Autodesk Fusion 360 part; units mm, degrees
(part 11 of 12)
  line L1843 (137.546, 134.2487) -> (141.8762, 136.7487)
  line L1844 (141.8762, 136.7487) -> (141.8762, 141.7487)
  line L1845 (141.8762, 141.7487) -> (137.546, 144.2487)
  line L1846 (148.2063, 144.2487) -> (143.8762, 141.7487)
  line L1847 (143.8762, 141.7487) -> (143.8762, 136.7487)
  line L1848 (143.8762, 136.7487) -> (148.2063, 134.2487)
  line L1849 (148.2063, 134.2487) -> (152.5364, 136.7487)
  line L1850 (152.5364, 136.7487) -> (152.5364, 141.7487)
  line L1851 (152.5364, 141.7487) -> (148.2063, 144.2487)
  line L1852 (-59.6687, 153.4808) -> (-63.9988, 150.9808)
  line L1853 (-63.9988, 150.9808) -> (-63.9988, 145.9808)
  line L1854 (-63.9988, 145.9808) -> (-59.6687, 143.4808)
  line L1855 (-59.6687, 143.4808) -> (-55.3385, 145.9808)
  line L1856 (-55.3385, 145.9808) -> (-55.3385, 150.9808)
  line L1857 (-55.3385, 150.9808) -> (-59.6687, 153.4808)
  line L1858 (-49.0084, 153.4808) -> (-53.3385, 150.9808)
  line L1859 (-53.3385, 150.9808) -> (-53.3385, 145.9808)
  line L1860 (-53.3385, 145.9808) -> (-49.0084, 143.4808)
  line L1861 (-49.0084, 143.4808) -> (-44.6783, 145.9808)
  line L1862 (-44.6783, 145.9808) -> (-44.6783, 150.9808)
  line L1863 (-44.6783, 150.9808) -> (-49.0084, 153.4808)
  line L1864 (-38.3482, 153.4808) -> (-42.6783, 150.9808)
  line L1865 (-42.6783, 150.9808) -> (-42.6783, 145.9808)
  line L1866 (-42.6783, 145.9808) -> (-38.3482, 143.4808)
  line L1867 (-38.3482, 143.4808) -> (-34.018, 145.9808)
  line L1868 (-34.018, 145.9808) -> (-34.018, 150.9808)
  line L1869 (-34.018, 150.9808) -> (-38.3482, 153.4808)
  line L1870 (-27.6879, 153.4808) -> (-32.018, 150.9808)
  line L1871 (-32.018, 150.9808) -> (-32.018, 145.9808)
  line L1872 (-32.018, 145.9808) -> (-27.6879, 143.4808)
  line L1873 (-27.6879, 143.4808) -> (-23.3578, 145.9808)
  line L1874 (-23.3578, 145.9808) -> (-23.3578, 150.9808)
  line L1875 (-23.3578, 150.9808) -> (-27.6879, 153.4808)
  line L1876 (-17.0277, 153.4808) -> (-21.3578, 150.9808)
  line L1877 (-21.3578, 150.9808) -> (-21.3578, 145.9808)
  line L1878 (-21.3578, 145.9808) -> (-17.0277, 143.4808)
  line L1879 (-17.0277, 143.4808) -> (-12.6975, 145.9808)
  line L1880 (-12.6975, 145.9808) -> (-12.6975, 150.9808)
  line L1881 (-12.6975, 150.9808) -> (-17.0277, 153.4808)
  line L1882 (-6.3674, 153.4808) -> (-10.6975, 150.9808)
  line L1883 (-10.6975, 150.9808) -> (-10.6975, 145.9808)
  line L1884 (-10.6975, 145.9808) -> (-6.3674, 143.4808)
  line L1885 (-6.3674, 143.4808) -> (-2.0373, 145.9808)
  line L1886 (-2.0373, 145.9808) -> (-2.0373, 150.9808)
  line L1887 (-2.0373, 150.9808) -> (-6.3674, 153.4808)
  line L1888 (4.2929, 153.4808) -> (-0.0373, 150.9808)
  line L1889 (-0.0373, 150.9808) -> (-0.0373, 145.9808)
  line L1890 (-0.0373, 145.9808) -> (4.2929, 143.4808)
  line L1891 (4.2929, 143.4808) -> (8.623, 145.9808)
  line L1892 (8.623, 145.9808) -> (8.623, 150.9808)
  line L1893 (8.623, 150.9808) -> (4.2929, 153.4808)
  line L1894 (14.9531, 153.4808) -> (10.623, 150.9808)
  line L1895 (10.623, 150.9808) -> (10.623, 145.9808)
  line L1896 (10.623, 145.9808) -> (14.9531, 143.4808)
  line L1897 (14.9531, 143.4808) -> (19.2832, 145.9808)
  line L1898 (19.2832, 145.9808) -> (19.2832, 150.9808)
  line L1899 (19.2832, 150.9808) -> (14.9531, 153.4808)
  line L1900 (25.6134, 153.4808) -> (21.2832, 150.9808)
  line L1901 (21.2832, 150.9808) -> (21.2832, 145.9808)
  line L1902 (21.2832, 145.9808) -> (25.6134, 143.4808)
  line L1903 (25.6134, 143.4808) -> (29.9435, 145.9808)
  line L1904 (29.9435, 145.9808) -> (29.9435, 150.9808)
  line L1905 (29.9435, 150.9808) -> (25.6134, 153.4808)
  line L1906 (36.2736, 153.4808) -> (31.9435, 150.9808)
  line L1907 (31.9435, 150.9808) -> (31.9435, 145.9808)
  line L1908 (31.9435, 145.9808) -> (36.2736, 143.4808)
  line L1909 (36.2736, 143.4808) -> (40.6037, 145.9808)
  line L1910 (40.6037, 145.9808) -> (40.6037, 150.9808)
  line L1911 (40.6037, 150.9808) -> (36.2736, 153.4808)
  line L1912 (46.9339, 153.4808) -> (42.6037, 150.9808)
  line L1913 (42.6037, 150.9808) -> (42.6037, 145.9808)
  line L1914 (42.6037, 145.9808) -> (46.9339, 143.4808)
  line L1915 (46.9339, 143.4808) -> (51.264, 145.9808)
  line L1916 (51.264, 145.9808) -> (51.264, 150.9808)
  line L1917 (51.264, 150.9808) -> (46.9339, 153.4808)
  line L1918 (57.5941, 153.4808) -> (53.264, 150.9808)
  line L1919 (53.264, 150.9808) -> (53.264, 145.9808)
  line L1920 (53.264, 145.9808) -> (57.5941, 143.4808)
  line L1921 (57.5941, 143.4808) -> (61.9242, 145.9808)
  line L1922 (61.9242, 145.9808) -> (61.9242, 150.9808)
  line L1923 (61.9242, 150.9808) -> (57.5941, 153.4808)
  line L1924 (68.2544, 153.4808) -> (63.9242, 150.9808)
  line L1925 (63.9242, 150.9808) -> (63.9242, 145.9808)
  line L1926 (63.9242, 145.9808) -> (68.2544, 143.4808)
  line L1927 (68.2544, 143.4808) -> (72.5845, 145.9808)
  line L1928 (72.5845, 145.9808) -> (72.5845, 150.9808)
  line L1929 (72.5845, 150.9808) -> (68.2544, 153.4808)
  line L1930 (78.9146, 153.4808) -> (74.5845, 150.9808)
  line L1931 (74.5845, 150.9808) -> (74.5845, 145.9808)
  line L1932 (74.5845, 145.9808) -> (78.9146, 143.4808)
  line L1933 (78.9146, 143.4808) -> (83.2448, 145.9808)
  line L1934 (83.2448, 145.9808) -> (83.2448, 150.9808)
  line L1935 (83.2448, 150.9808) -> (78.9146, 153.4808)
  line L1936 (89.5749, 153.4808) -> (85.2448, 150.9808)
  line L1937 (85.2448, 150.9808) -> (85.2448, 145.9808)
  line L1938 (85.2448, 145.9808) -> (89.5749, 143.4808)
  line L1939 (89.5749, 143.4808) -> (93.905, 145.9808)
  line L1940 (93.905, 145.9808) -> (93.905, 150.9808)
  line L1941 (93.905, 150.9808) -> (89.5749, 153.4808)
  line L1942 (100.2351, 153.4808) -> (95.905, 150.9808)
  line L1943 (95.905, 150.9808) -> (95.905, 145.9808)
  line L1944 (95.905, 145.9808) -> (100.2351, 143.4808)
  line L1945 (100.2351, 143.4808) -> (104.5653, 145.9808)
  line L1946 (104.5653, 145.9808) -> (104.5653, 150.9808)
  line L1947 (104.5653, 150.9808) -> (100.2351, 153.4808)
  line L1948 (110.8954, 153.4808) -> (106.5653, 150.9808)
  line L1949 (106.5653, 150.9808) -> (106.5653, 145.9808)
  line L1950 (106.5653, 145.9808) -> (110.8954, 143.4808)
  line L1951 (110.8954, 143.4808) -> (115.2255, 145.9808)
  line L1952 (115.2255, 145.9808) -> (115.2255, 150.9808)
  line L1953 (115.2255, 150.9808) -> (110.8954, 153.4808)
  line L1954 (121.5556, 153.4808) -> (117.2255, 150.9808)
  line L1955 (117.2255, 150.9808) -> (117.2255, 145.9808)
  line L1956 (117.2255, 145.9808) -> (121.5556, 143.4808)
  line L1957 (121.5556, 143.4808) -> (125.8858, 145.9808)
  line L1958 (125.8858, 145.9808) -> (125.8858, 150.9808)
  line L1959 (125.8858, 150.9808) -> (121.5556, 153.4808)
  line L1960 (132.2159, 153.4808) -> (127.8858, 150.9808)
  line L1961 (127.8858, 150.9808) -> (127.8858, 145.9808)
  line L1962 (127.8858, 145.9808) -> (132.2159, 143.4808)
  line L1963 (132.2159, 143.4808) -> (136.546, 145.9808)
  line L1964 (136.546, 145.9808) -> (136.546, 150.9808)
  line L1965 (136.546, 150.9808) -> (132.2159, 153.4808)
  line L1966 (142.8762, 153.4808) -> (138.546, 150.9808)
  line L1967 (138.546, 150.9808) -> (138.546, 145.9808)
  line L1968 (138.546, 145.9808) -> (142.8762, 143.4808)
  line L1969 (142.8762, 143.4808) -> (147.2063, 145.9808)
  line L1970 (147.2063, 145.9808) -> (147.2063, 150.9808)
  line L1971 (147.2063, 150.9808) -> (142.8762, 153.4808)
  line L1972 (-64.9988, 162.7128) -> (-69.3289, 160.2128)
  line L1973 (-69.3289, 160.2128) -> (-69.3289, 155.2128)
  line L1974 (-69.3289, 155.2128) -> (-64.9988, 152.7128)
  line L1975 (-64.9988, 152.7128) -> (-60.6687, 155.2128)
  line L1976 (-60.6687, 155.2128) -> (-60.6687, 160.2128)
  line L1977 (-60.6687, 160.2128) -> (-64.9988, 162.7128)
  line L1978 (-54.3385, 162.7128) -> (-58.6687, 160.2128)
  line L1979 (-58.6687, 160.2128) -> (-58.6687, 155.2128)
  line L1980 (-58.6687, 155.2128) -> (-54.3385, 152.7128)
  line L1981 (-54.3385, 152.7128) -> (-50.0084, 155.2128)
  line L1982 (-50.0084, 155.2128) -> (-50.0084, 160.2128)
  line L1983 (-50.0084, 160.2128) -> (-54.3385, 162.7128)
  line L1984 (-43.6783, 162.7128) -> (-48.0084, 160.2128)
  line L1985 (-48.0084, 160.2128) -> (-48.0084, 155.2128)
  line L1986 (-48.0084, 155.2128) -> (-43.6783, 152.7128)
  line L1987 (-43.6783, 152.7128) -> (-39.3482, 155.2128)
  line L1988 (-39.3482, 155.2128) -> (-39.3482, 160.2128)
  line L1989 (-39.3482, 160.2128) -> (-43.6783, 162.7128)
  line L1990 (-33.018, 162.7128) -> (-37.3482, 160.2128)
  line L1991 (-37.3482, 160.2128) -> (-37.3482, 155.2128)
  line L1992 (-37.3482, 155.2128) -> (-33.018, 152.7128)
  line L1993 (-33.018, 152.7128) -> (-28.6879, 155.2128)
  line L1994 (-28.6879, 155.2128) -> (-28.6879, 160.2128)
  line L1995 (-28.6879, 160.2128) -> (-33.018, 162.7128)
  line L1996 (-22.3578, 162.7128) -> (-26.6879, 160.2128)
  line L1997 (-26.6879, 160.2128) -> (-26.6879, 155.2128)
  line L1998 (-26.6879, 155.2128) -> (-22.3578, 152.7128)
  line L1999 (-22.3578, 152.7128) -> (-18.0277, 155.2128)
  line L2000 (-18.0277, 155.2128) -> (-18.0277, 160.2128)
  line L2001 (-18.0277, 160.2128) -> (-22.3578, 162.7128)
  line L2002 (-11.6975, 162.7128) -> (-16.0277, 160.2128)
  line L2003 (-16.0277, 160.2128) -> (-16.0277, 155.2128)
  line L2004 (-16.0277, 155.2128) -> (-11.6975, 152.7128)
  line L2005 (-11.6975, 152.7128) -> (-7.3674, 155.2128)
  line L2006 (-7.3674, 155.2128) -> (-7.3674, 160.2128)
  line L2007 (-7.3674, 160.2128) -> (-11.6975, 162.7128)
  line L2008 (-1.0373, 162.7128) -> (-5.3674, 160.2128)
  line L2009 (-5.3674, 160.2128) -> (-5.3674, 155.2128)
  line L2010 (-5.3674, 155.2128) -> (-1.0373, 152.7128)
  line L2011 (-1.0373, 152.7128) -> (3.2929, 155.2128)
  line L2012 (3.2929, 155.2128) -> (3.2929, 160.2128)
  line L2013 (3.2929, 160.2128) -> (-1.0373, 162.7128)
  line L2014 (9.623, 162.7128) -> (5.2929, 160.2128)
  line L2015 (5.2929, 160.2128) -> (5.2929, 155.2128)
  line L2016 (5.2929, 155.2128) -> (9.623, 152.7128)
  line L2017 (9.623, 152.7128) -> (13.9531, 155.2128)
  line L2018 (13.9531, 155.2128) -> (13.9531, 160.2128)
  line L2019 (13.9531, 160.2128) -> (9.623, 162.7128)
  line L2020 (20.2832, 162.7128) -> (15.9531, 160.2128)
  line L2021 (15.9531, 160.2128) -> (15.9531, 155.2128)
  line L2022 (15.9531, 155.2128) -> (20.2832, 152.7128)
  line L2023 (20.2832, 152.7128) -> (24.6134, 155.2128)
  line L2024 (24.6134, 155.2128) -> (24.6134, 160.2128)
  line L2025 (24.6134, 160.2128) -> (20.2832, 162.7128)
  line L2026 (30.9435, 162.7128) -> (26.6134, 160.2128)
  line L2027 (26.6134, 160.2128) -> (26.6134, 155.2128)
  line L2028 (26.6134, 155.2128) -> (30.9435, 152.7128)
  line L2029 (30.9435, 152.7128) -> (35.2736, 155.2128)
  line L2030 (35.2736, 155.2128) -> (35.2736, 160.2128)
  line L2031 (35.2736, 160.2128) -> (30.9435, 162.7128)
  line L2032 (41.6037, 162.7128) -> (37.2736, 160.2128)
  line L2033 (37.2736, 160.2128) -> (37.2736, 155.2128)
  line L2034 (37.2736, 155.2128) -> (41.6037, 152.7128)
  line L2035 (41.6037, 152.7128) -> (45.9339, 155.2128)
  line L2036 (45.9339, 155.2128) -> (45.9339, 160.2128)
  line L2037 (45.9339, 160.2128) -> (41.6037, 162.7128)
  line L2038 (52.264, 162.7128) -> (47.9339, 160.2128)
  line L2039 (47.9339, 160.2128) -> (47.9339, 155.2128)
  line L2040 (47.9339, 155.2128) -> (52.264, 152.7128)
  line L2041 (52.264, 152.7128) -> (56.5941, 155.2128)
  line L2042 (56.5941, 155.2128) -> (56.5941, 160.2128)
  line L2043 (56.5941, 160.2128) -> (52.264, 162.7128)
  line L2044 (62.9242, 162.7128) -> (58.5941, 160.2128)
  line L2045 (58.5941, 160.2128) -> (58.5941, 155.2128)
  line L2046 (58.5941, 155.2128) -> (62.9242, 152.7128)
  line L2047 (62.9242, 152.7128) -> (67.2544, 155.2128)
  line L2048 (67.2544, 155.2128) -> (67.2544, 160.2128)
  line L2049 (67.2544, 160.2128) -> (62.9242, 162.7128)
  line L2050 (73.5845, 162.7128) -> (69.2544, 160.2128)
  line L2051 (69.2544, 160.2128) -> (69.2544, 155.2128)
  line L2052 (69.2544, 155.2128) -> (73.5845, 152.7128)
  line L2053 (73.5845, 152.7128) -> (77.9146, 155.2128)
  line L2054 (77.9146, 155.2128) -> (77.9146, 160.2128)
  line L2055 (77.9146, 160.2128) -> (73.5845, 162.7128)
  line L2056 (84.2448, 162.7128) -> (79.9146, 160.2128)
  line L2057 (79.9146, 160.2128) -> (79.9146, 155.2128)
  line L2058 (79.9146, 155.2128) -> (84.2448, 152.7128)
  line L2059 (84.2448, 152.7128) -> (88.5749, 155.2128)
  line L2060 (88.5749, 155.2128) -> (88.5749, 160.2128)
  line L2061 (88.5749, 160.2128) -> (84.2448, 162.7128)
  line L2062 (94.905, 162.7128) -> (90.5749, 160.2128)
  line L2063 (90.5749, 160.2128) -> (90.5749, 155.2128)
  line L2064 (90.5749, 155.2128) -> (94.905, 152.7128)
  line L2065 (94.905, 152.7128) -> (99.2351, 155.2128)
  line L2066 (99.2351, 155.2128) -> (99.2351, 160.2128)
  line L2067 (99.2351, 160.2128) -> (94.905, 162.7128)
  line L2068 (105.5653, 162.7128) -> (101.2351, 160.2128)
  line L2069 (101.2351, 160.2128) -> (101.2351, 155.2128)
  line L2070 (101.2351, 155.2128) -> (105.5653, 152.7128)
  line L2071 (105.5653, 152.7128) -> (109.8954, 155.2128)
  line L2072 (109.8954, 155.2128) -> (109.8954, 160.2128)
  line L2073 (109.8954, 160.2128) -> (105.5653, 162.7128)
  line L2074 (116.2255, 162.7128) -> (111.8954, 160.2128)
  line L2075 (111.8954, 160.2128) -> (111.8954, 155.2128)
  line L2076 (111.8954, 155.2128) -> (116.2255, 152.7128)
  line L2077 (116.2255, 152.7128) -> (120.5556, 155.2128)
  line L2078 (120.5556, 155.2128) -> (120.5556, 160.2128)
  line L2079 (120.5556, 160.2128) -> (116.2255, 162.7128)
  line L2080 (126.8858, 162.7128) -> (122.5556, 160.2128)
  line L2081 (122.5556, 160.2128) -> (122.5556, 155.2128)
  line L2082 (122.5556, 155.2128) -> (126.8858, 152.7128)
  line L2083 (126.8858, 152.7128) -> (131.2159, 155.2128)
  line L2084 (131.2159, 155.2128) -> (131.2159, 160.2128)
  line L2085 (131.2159, 160.2128) -> (126.8858, 162.7128)
  line L2086 (137.546, 162.7128) -> (133.2159, 160.2128)
  line L2087 (133.2159, 160.2128) -> (133.2159, 155.2128)
  line L2088 (133.2159, 155.2128) -> (137.546, 152.7128)
  line L2089 (137.546, 152.7128) -> (141.8762, 155.2128)
  line L2090 (141.8762, 155.2128) -> (141.8762, 160.2128)
  line L2091 (141.8762, 160.2128) -> (137.546, 162.7128)
  line L2092 (148.2063, 162.7128) -> (143.8762, 160.2128)
  line L2093 (143.8762, 160.2128) -> (143.8762, 155.2128)
  line L2094 (143.8762, 155.2128) -> (148.2063, 152.7128)
  line L2095 (148.2063, 152.7128) -> (152.5364, 155.2128)
  line L2096 (152.5364, 155.2128) -> (152.5364, 160.2128)
  line L2097 (152.5364, 160.2128) -> (148.2063, 162.7128)
  line L2098 (-59.6687, 171.9449) -> (-63.9988, 169.4449)
  line L2099 (-63.9988, 169.4449) -> (-63.9988, 164.4449)
  line L2100 (-63.9988, 164.4449) -> (-59.6687, 161.9449)
  line L2101 (-59.6687, 161.9449) -> (-55.3385, 164.4449)
  line L2102 (-55.3385, 164.4449) -> (-55.3385, 169.4449)
  line L2103 (-55.3385, 169.4449) -> (-59.6687, 171.9449)
  line L2104 (-49.0084, 171.9449) -> (-53.3385, 169.4449)
  line L2105 (-53.3385, 169.4449) -> (-53.3385, 164.4449)
  line L2106 (-53.3385, 164.4449) -> (-49.0084, 161.9449)
  line L2107 (-49.0084, 161.9449) -> (-44.6783, 164.4449)
  line L2108 (-44.6783, 164.4449) -> (-44.6783, 169.4449)
  line L2109 (-44.6783, 169.4449) -> (-49.0084, 171.9449)
  line L2110 (-38.3482, 171.9449) -> (-42.6783, 169.4449)
  line L2111 (-42.6783, 169.4449) -> (-42.6783, 164.4449)
  line L2112 (-42.6783, 164.4449) -> (-38.3482, 161.9449)
  line L2113 (-38.3482, 161.9449) -> (-34.018, 164.4449)
  line L2114 (-34.018, 164.4449) -> (-34.018, 169.4449)
  line L2115 (-34.018, 169.4449) -> (-38.3482, 171.9449)
  line L2116 (-27.6879, 171.9449) -> (-32.018, 169.4449)
  line L2117 (-32.018, 169.4449) -> (-32.018, 164.4449)
  line L2118 (-32.018, 164.4449) -> (-27.6879, 161.9449)
  line L2119 (-27.6879, 161.9449) -> (-23.3578, 164.4449)
  line L2120 (-23.3578, 164.4449) -> (-23.3578, 169.4449)
  line L2121 (-23.3578, 169.4449) -> (-27.6879, 171.9449)
  line L2122 (-17.0277, 171.9449) -> (-21.3578, 169.4449)
  line L2123 (-21.3578, 169.4449) -> (-21.3578, 164.4449)
  line L2124 (-21.3578, 164.4449) -> (-17.0277, 161.9449)
  line L2125 (-17.0277, 161.9449) -> (-12.6975, 164.4449)
  line L2126 (-12.6975, 164.4449) -> (-12.6975, 169.4449)
  line L2127 (-12.6975, 169.4449) -> (-17.0277, 171.9449)
  line L2128 (-6.3674, 171.9449) -> (-10.6975, 169.4449)
  line L2129 (-10.6975, 169.4449) -> (-10.6975, 164.4449)
  line L2130 (-10.6975, 164.4449) -> (-6.3674, 161.9449)
  line L2131 (-6.3674, 161.9449) -> (-2.0373, 164.4449)
  line L2132 (-2.0373, 164.4449) -> (-2.0373, 169.4449)
  line L2133 (-2.0373, 169.4449) -> (-6.3674, 171.9449)
  line L2134 (4.2929, 171.9449) -> (-0.0373, 169.4449)
  line L2135 (-0.0373, 169.4449) -> (-0.0373, 164.4449)
  line L2136 (-0.0373, 164.4449) -> (4.2929, 161.9449)
  line L2137 (4.2929, 161.9449) -> (8.623, 164.4449)
  line L2138 (8.623, 164.4449) -> (8.623, 169.4449)
  line L2139 (8.623, 169.4449) -> (4.2929, 171.9449)
  line L2140 (14.9531, 171.9449) -> (10.623, 169.4449)
  line L2141 (10.623, 169.4449) -> (10.623, 164.4449)
  line L2142 (10.623, 164.4449) -> (14.9531, 161.9449)
  line L2143 (14.9531, 161.9449) -> (19.2832, 164.4449)
  line L2144 (19.2832, 164.4449) -> (19.2832, 169.4449)
  line L2145 (19.2832, 169.4449) -> (14.9531, 171.9449)
  line L2146 (25.6134, 171.9449) -> (21.2832, 169.4449)
  line L2147 (21.2832, 169.4449) -> (21.2832, 164.4449)
  line L2148 (21.2832, 164.4449) -> (25.6134, 161.9449)
  line L2149 (25.6134, 161.9449) -> (29.9435, 164.4449)
  line L2150 (29.9435, 164.4449) -> (29.9435, 169.4449)
  line L2151 (29.9435, 169.4449) -> (25.6134, 171.9449)
  line L2152 (36.2736, 171.9449) -> (31.9435, 169.4449)
  line L2153 (31.9435, 169.4449) -> (31.9435, 164.4449)
  line L2154 (31.9435, 164.4449) -> (36.2736, 161.9449)
  line L2155 (36.2736, 161.9449) -> (40.6037, 164.4449)
  line L2156 (40.6037, 164.4449) -> (40.6037, 169.4449)
  line L2157 (40.6037, 169.4449) -> (36.2736, 171.9449)
  line L2158 (46.9339, 171.9449) -> (42.6037, 169.4449)
  line L2159 (42.6037, 169.4449) -> (42.6037, 164.4449)
  line L2160 (42.6037, 164.4449) -> (46.9339, 161.9449)
  line L2161 (46.9339, 161.9449) -> (51.264, 164.4449)
  line L2162 (51.264, 164.4449) -> (51.264, 169.4449)
  line L2163 (51.264, 169.4449) -> (46.9339, 171.9449)
  line L2164 (57.5941, 171.9449) -> (53.264, 169.4449)
  line L2165 (53.264, 169.4449) -> (53.264, 164.4449)
  line L2166 (53.264, 164.4449) -> (57.5941, 161.9449)
  line L2167 (57.5941, 161.9449) -> (61.9242, 164.4449)
  line L2168 (61.9242, 164.4449) -> (61.9242, 169.4449)
  line L2169 (61.9242, 169.4449) -> (57.5941, 171.9449)
  line L2170 (68.2544, 171.9449) -> (63.9242, 169.4449)
  line L2171 (63.9242, 169.4449) -> (63.9242, 164.4449)
  line L2172 (63.9242, 164.4449) -> (68.2544, 161.9449)
  line L2173 (68.2544, 161.9449) -> (72.5845, 164.4449)
  line L2174 (72.5845, 164.4449) -> (72.5845, 169.4449)
  line L2175 (72.5845, 169.4449) -> (68.2544, 171.9449)
  line L2176 (78.9146, 171.9449) -> (74.5845, 169.4449)
  line L2177 (74.5845, 169.4449) -> (74.5845, 164.4449)
  line L2178 (74.5845, 164.4449) -> (78.9146, 161.9449)
  line L2179 (78.9146, 161.9449) -> (83.2448, 164.4449)
  line L2180 (83.2448, 164.4449) -> (83.2448, 169.4449)
  line L2181 (83.2448, 169.4449) -> (78.9146, 171.9449)
  line L2182 (89.5749, 171.9449) -> (85.2448, 169.4449)
  line L2183 (85.2448, 169.4449) -> (85.2448, 164.4449)
  line L2184 (85.2448, 164.4449) -> (89.5749, 161.9449)
  line L2185 (89.5749, 161.9449) -> (93.905, 164.4449)
  line L2186 (93.905, 164.4449) -> (93.905, 169.4449)
  line L2187 (93.905, 169.4449) -> (89.5749, 171.9449)
  line L2188 (100.2351, 171.9449) -> (95.905, 169.4449)
  line L2189 (95.905, 169.4449) -> (95.905, 164.4449)
  line L2190 (95.905, 164.4449) -> (100.2351, 161.9449)
  line L2191 (100.2351, 161.9449) -> (104.5653, 164.4449)
  line L2192 (104.5653, 164.4449) -> (104.5653, 169.4449)
  line L2193 (104.5653, 169.4449) -> (100.2351, 171.9449)
  line L2194 (110.8954, 171.9449) -> (106.5653, 169.4449)
  line L2195 (106.5653, 169.4449) -> (106.5653, 164.4449)
  line L2196 (106.5653, 164.4449) -> (110.8954, 161.9449)
  line L2197 (110.8954, 161.9449) -> (115.2255, 164.4449)
  line L2198 (115.2255, 164.4449) -> (115.2255, 169.4449)
  line L2199 (115.2255, 169.4449) -> (110.8954, 171.9449)
  line L2200 (121.5556, 171.9449) -> (117.2255, 169.4449)
  line L2201 (117.2255, 169.4449) -> (117.2255, 164.4449)
  line L2202 (117.2255, 164.4449) -> (121.5556, 161.9449)
  line L2203 (121.5556, 161.9449) -> (125.8858, 164.4449)
  line L2204 (125.8858, 164.4449) -> (125.8858, 169.4449)
  line L2205 (125.8858, 169.4449) -> (121.5556, 171.9449)
  line L2206 (132.2159, 171.9449) -> (127.8858, 169.4449)
  line L2207 (127.8858, 169.4449) -> (127.8858, 164.4449)
  line L2208 (127.8858, 164.4449) -> (132.2159, 161.9449)
  line L2209 (132.2159, 161.9449) -> (136.546, 164.4449)
  line L2210 (136.546, 164.4449) -> (136.546, 169.4449)
  line L2211 (136.546, 169.4449) -> (132.2159, 171.9449)
  line L2212 (142.8762, 171.9449) -> (138.546, 169.4449)
  line L2213 (138.546, 169.4449) -> (138.546, 164.4449)
  line L2214 (138.546, 164.4449) -> (142.8762, 161.9449)
  line L2215 (142.8762, 161.9449) -> (147.2063, 164.4449)
  line L2216 (147.2063, 164.4449) -> (147.2063, 169.4449)
  line L2217 (147.2063, 169.4449) -> (142.8762, 171.9449)
  line L2218 (-64.9988, 181.1769) -> (-69.3289, 178.6769)
  line L2219 (-69.3289, 178.6769) -> (-69.3289, 173.6769)
  line L2220 (-69.3289, 173.6769) -> (-64.9988, 171.1769)
  line L2221 (-64.9988, 171.1769) -> (-60.6687, 173.6769)
  line L2222 (-60.6687, 173.6769) -> (-60.6687, 178.6769)
  line L2223 (-60.6687, 178.6769) -> (-64.9988, 181.1769)
  line L2224 (-54.3385, 181.1769) -> (-58.6687, 178.6769)
  line L2225 (-58.6687, 178.6769) -> (-58.6687, 173.6769)
  line L2226 (-58.6687, 173.6769) -> (-54.3385, 171.1769)
  line L2227 (-54.3385, 171.1769) -> (-50.0084, 173.6769)
  line L2228 (-50.0084, 173.6769) -> (-50.0084, 178.6769)
  line L2229 (-50.0084, 178.6769) -> (-54.3385, 181.1769)
  line L2230 (-43.6783, 181.1769) -> (-48.0084, 178.6769)
  line L2231 (-48.0084, 178.6769) -> (-48.0084, 173.6769)
  line L2232 (-48.0084, 173.6769) -> (-43.6783, 171.1769)
  line L2233 (-43.6783, 171.1769) -> (-39.3482, 173.6769)
  line L2234 (-39.3482, 173.6769) -> (-39.3482, 178.6769)
  line L2235 (-39.3482, 178.6769) -> (-43.6783, 181.1769)
  line L2236 (-33.018, 181.1769) -> (-37.3482, 178.6769)
  line L2237 (-37.3482, 178.6769) -> (-37.3482, 173.6769)
  line L2238 (-37.3482, 173.6769) -> (-33.018, 171.1769)
  line L2239 (-33.018, 171.1769) -> (-28.6879, 173.6769)
  line L2240 (-28.6879, 173.6769) -> (-28.6879, 178.6769)
  line L2241 (-28.6879, 178.6769) -> (-33.018, 181.1769)
  line L2242 (-22.3578, 181.1769) -> (-26.6879, 178.6769)
  line L2243 (-26.6879, 178.6769) -> (-26.6879, 173.6769)
  line L2244 (-26.6879, 173.6769) -> (-22.3578, 171.1769)
  line L2245 (-22.3578, 171.1769) -> (-18.0277, 173.6769)
  line L2246 (-18.0277, 173.6769) -> (-18.0277, 178.6769)
  line L2247 (-18.0277, 178.6769) -> (-22.3578, 181.1769)
  line L2248 (-11.6975, 181.1769) -> (-16.0277, 178.6769)
  line L2249 (-16.0277, 178.6769) -> (-16.0277, 173.6769)
  line L2250 (-16.0277, 173.6769) -> (-11.6975, 171.1769)
  line L2251 (-11.6975, 171.1769) -> (-7.3674, 173.6769)
  line L2252 (-7.3674, 173.6769) -> (-7.3674, 178.6769)
  line L2253 (-7.3674, 178.6769) -> (-11.6975, 181.1769)
  line L2254 (-1.0373, 181.1769) -> (-5.3674, 178.6769)
  line L2255 (-5.3674, 178.6769) -> (-5.3674, 173.6769)
  line L2256 (-5.3674, 173.6769) -> (-1.0373, 171.1769)
  line L2257 (-1.0373, 171.1769) -> (3.2929, 173.6769)
  line L2258 (3.2929, 173.6769) -> (3.2929, 178.6769)
  line L2259 (3.2929, 178.6769) -> (-1.0373, 181.1769)
  line L2260 (9.623, 181.1769) -> (5.2929, 178.6769)
  line L2261 (5.2929, 178.6769) -> (5.2929, 173.6769)
  line L2262 (5.2929, 173.6769) -> (9.623, 171.1769)
  line L2263 (9.623, 171.1769) -> (13.9531, 173.6769)
  line L2264 (13.9531, 173.6769) -> (13.9531, 178.6769)
  line L2265 (13.9531, 178.6769) -> (9.623, 181.1769)
  line L2266 (20.2832, 181.1769) -> (15.9531, 178.6769)
  line L2267 (15.9531, 178.6769) -> (15.9531, 173.6769)
  line L2268 (15.9531, 173.6769) -> (20.2832, 171.1769)
  line L2269 (20.2832, 171.1769) -> (24.6134, 173.6769)
  line L2270 (24.6134, 173.6769) -> (24.6134, 178.6769)
  line L2271 (24.6134, 178.6769) -> (20.2832, 181.1769)
  line L2272 (30.9435, 181.1769) -> (26.6134, 178.6769)
  line L2273 (26.6134, 178.6769) -> (26.6134, 173.6769)
  line L2274 (26.6134, 173.6769) -> (30.9435, 171.1769)
  line L2275 (30.9435, 171.1769) -> (35.2736, 173.6769)
  line L2276 (35.2736, 173.6769) -> (35.2736, 178.6769)
  line L2277 (35.2736, 178.6769) -> (30.9435, 181.1769)
  line L2278 (41.6037, 181.1769) -> (37.2736, 178.6769)
  line L2279 (37.2736, 178.6769) -> (37.2736, 173.6769)
  line L2280 (37.2736, 173.6769) -> (41.6037, 171.1769)
  line L2281 (41.6037, 171.1769) -> (45.9339, 173.6769)
  line L2282 (45.9339, 173.6769) -> (45.9339, 178.6769)
  line L2283 (45.9339, 178.6769) -> (41.6037, 181.1769)
  line L2284 (52.264, 181.1769) -> (47.9339, 178.6769)
  line L2285 (47.9339, 178.6769) -> (47.9339, 173.6769)
  line L2286 (47.9339, 173.6769) -> (52.264, 171.1769)
  line L2287 (52.264, 171.1769) -> (56.5941, 173.6769)
  line L2288 (56.5941, 173.6769) -> (56.5941, 178.6769)
  line L2289 (56.5941, 178.6769) -> (52.264, 181.1769)
  line L2290 (62.9242, 181.1769) -> (58.5941, 178.6769)
  line L2291 (58.5941, 178.6769) -> (58.5941, 173.6769)
  line L2292 (58.5941, 173.6769) -> (62.9242, 171.1769)
  line L2293 (62.9242, 171.1769) -> (67.2544, 173.6769)
  line L2294 (67.2544, 173.6769) -> (67.2544, 178.6769)
  line L2295 (67.2544, 178.6769) -> (62.9242, 181.1769)
  line L2296 (73.5845, 181.1769) -> (69.2544, 178.6769)
  line L2297 (69.2544, 178.6769) -> (69.2544, 173.6769)
  line L2298 (69.2544, 173.6769) -> (73.5845, 171.1769)
  line L2299 (73.5845, 171.1769) -> (77.9146, 173.6769)
  line L2300 (77.9146, 173.6769) -> (77.9146, 178.6769)
  line L2301 (77.9146, 178.6769) -> (73.5845, 181.1769)
  line L2302 (84.2448, 181.1769) -> (79.9146, 178.6769)
  line L2303 (79.9146, 178.6769) -> (79.9146, 173.6769)
  line L2304 (79.9146, 173.6769) -> (84.2448, 171.1769)
  line L2305 (84.2448, 171.1769) -> (88.5749, 173.6769)
  line L2306 (88.5749, 173.6769) -> (88.5749, 178.6769)
  line L2307 (88.5749, 178.6769) -> (84.2448, 181.1769)
  line L2308 (94.905, 181.1769) -> (90.5749, 178.6769)
  line L2309 (90.5749, 178.6769) -> (90.5749, 173.6769)
  line L2310 (90.5749, 173.6769) -> (94.905, 171.1769)
  line L2311 (94.905, 171.1769) -> (99.2351, 173.6769)
  line L2312 (99.2351, 173.6769) -> (99.2351, 178.6769)
  line L2313 (99.2351, 178.6769) -> (94.905, 181.1769)
  line L2314 (105.5653, 181.1769) -> (101.2351, 178.6769)
  line L2315 (101.2351, 178.6769) -> (101.2351, 173.6769)
  line L2316 (101.2351, 173.6769) -> (105.5653, 171.1769)
  line L2317 (105.5653, 171.1769) -> (109.8954, 173.6769)
  line L2318 (109.8954, 173.6769) -> (109.8954, 178.6769)
  line L2319 (109.8954, 178.6769) -> (105.5653, 181.1769)
  line L2320 (116.2255, 181.1769) -> (111.8954, 178.6769)
  line L2321 (111.8954, 178.6769) -> (111.8954, 173.6769)
  line L2322 (111.8954, 173.6769) -> (116.2255, 171.1769)
  line L2323 (116.2255, 171.1769) -> (120.5556, 173.6769)
  line L2324 (120.5556, 173.6769) -> (120.5556, 178.6769)
  line L2325 (120.5556, 178.6769) -> (116.2255, 181.1769)
  line L2326 (126.8858, 181.1769) -> (122.5556, 178.6769)
  line L2327 (122.5556, 178.6769) -> (122.5556, 173.6769)
  line L2328 (122.5556, 173.6769) -> (126.8858, 171.1769)
  line L2329 (126.8858, 171.1769) -> (131.2159, 173.6769)
  line L2330 (131.2159, 173.6769) -> (131.2159, 178.6769)
  line L2331 (131.2159, 178.6769) -> (126.8858, 181.1769)
  line L2332 (137.546, 181.1769) -> (133.2159, 178.6769)
  line L2333 (133.2159, 178.6769) -> (133.2159, 173.6769)
  line L2334 (133.2159, 173.6769) -> (137.546, 171.1769)
  line L2335 (137.546, 171.1769) -> (141.8762, 173.6769)
  line L2336 (141.8762, 173.6769) -> (141.8762, 178.6769)
  line L2337 (141.8762, 178.6769) -> (137.546, 181.1769)
  line L2338 (148.2063, 181.1769) -> (143.8762, 178.6769)
  line L2339 (143.8762, 178.6769) -> (143.8762, 173.6769)
  line L2340 (143.8762, 173.6769) -> (148.2063, 171.1769)
  line L2341 (148.2063, 171.1769) -> (152.5364, 173.6769)
  line L2342 (152.5364, 173.6769) -> (152.5364, 178.6769)
  line L2343 (152.5364, 178.6769) -> (148.2063, 181.1769)
  line L2344 (-59.6687, 190.409) -> (-63.9988, 187.909)
  line L2345 (-63.9988, 187.909) -> (-63.9988, 182.909)
  line L2346 (-63.9988, 182.909) -> (-59.6687, 180.409)
  line L2347 (-59.6687, 180.409) -> (-55.3385, 182.909)
  line L2348 (-55.3385, 182.909) -> (-55.3385, 187.909)
  line L2349 (-55.3385, 187.909) -> (-59.6687, 190.409)
  line L2350 (-49.0084, 190.409) -> (-53.3385, 187.909)
  line L2351 (-53.3385, 187.909) -> (-53.3385, 182.909)
  line L2352 (-53.3385, 182.909) -> (-49.0084, 180.409)
  line L2353 (-49.0084, 180.409) -> (-44.6783, 182.909)
  line L2354 (-44.6783, 182.909) -> (-44.6783, 187.909)
  line L2355 (-44.6783, 187.909) -> (-49.0084, 190.409)
  line L2356 (-38.3482, 190.409) -> (-42.6783, 187.909)
  line L2357 (-42.6783, 187.909) -> (-42.6783, 182.909)
  line L2358 (-42.6783, 182.909) -> (-38.3482, 180.409)
  line L2359 (-38.3482, 180.409) -> (-34.018, 182.909)
  line L2360 (-34.018, 182.909) -> (-34.018, 187.909)
  line L2361 (-34.018, 187.909) -> (-38.3482, 190.409)
  line L2362 (-27.6879, 190.409) -> (-32.018, 187.909)
  line L2363 (-32.018, 187.909) -> (-32.018, 182.909)
  line L2364 (-32.018, 182.909) -> (-27.6879, 180.409)
  line L2365 (-27.6879, 180.409) -> (-23.3578, 182.909)
  line L2366 (-23.3578, 182.909) -> (-23.3578, 187.909)
  line L2367 (-23.3578, 187.909) -> (-27.6879, 190.409)
  line L2368 (-17.0277, 190.409) -> (-21.3578, 187.909)
  line L2369 (-21.3578, 187.909) -> (-21.3578, 182.909)
  line L2370 (-21.3578, 182.909) -> (-17.0277, 180.409)
  line L2371 (-17.0277, 180.409) -> (-12.6975, 182.909)
  line L2372 (-12.6975, 182.909) -> (-12.6975, 187.909)
  line L2373 (-12.6975, 187.909) -> (-17.0277, 190.409)
  line L2374 (-6.3674, 190.409) -> (-10.6975, 187.909)
  line L2375 (-10.6975, 187.909) -> (-10.6975, 182.909)
  line L2376 (-10.6975, 182.909) -> (-6.3674, 180.409)
  line L2377 (-6.3674, 180.409) -> (-2.0373, 182.909)
  line L2378 (-2.0373, 182.909) -> (-2.0373, 187.909)
  line L2379 (-2.0373, 187.909) -> (-6.3674, 190.409)
  line L2380 (4.2929, 190.409) -> (-0.0373, 187.909)
  line L2381 (-0.0373, 187.909) -> (-0.0373, 182.909)
  line L2382 (-0.0373, 182.909) -> (4.2929, 180.409)
  line L2383 (4.2929, 180.409) -> (8.623, 182.909)
  line L2384 (8.623, 182.909) -> (8.623, 187.909)
  line L2385 (8.623, 187.909) -> (4.2929, 190.409)
  line L2386 (14.9531, 190.409) -> (10.623, 187.909)
  line L2387 (10.623, 187.909) -> (10.623, 182.909)
  line L2388 (10.623, 182.909) -> (14.9531, 180.409)
  line L2389 (14.9531, 180.409) -> (19.2832, 182.909)
  line L2390 (19.2832, 182.909) -> (19.2832, 187.909)
  line L2391 (19.2832, 187.909) -> (14.9531, 190.409)
  line L2392 (25.6134, 190.409) -> (21.2832, 187.909)
  line L2393 (21.2832, 187.909) -> (21.2832, 182.909)
  line L2394 (21.2832, 182.909) -> (25.6134, 180.409)
  line L2395 (25.6134, 180.409) -> (29.9435, 182.909)
  line L2396 (29.9435, 182.909) -> (29.9435, 187.909)
  line L2397 (29.9435, 187.909) -> (25.6134, 190.409)
  line L2398 (36.2736, 190.409) -> (31.9435, 187.909)
  line L2399 (31.9435, 187.909) -> (31.9435, 182.909)
  line L2400 (31.9435, 182.909) -> (36.2736, 180.409)
  line L2401 (36.2736, 180.409) -> (40.6037, 182.909)
  line L2402 (40.6037, 182.909) -> (40.6037, 187.909)
  line L2403 (40.6037, 187.909) -> (36.2736, 190.409)
  line L2404 (46.9339, 190.409) -> (42.6037, 187.909)
  line L2405 (42.6037, 187.909) -> (42.6037, 182.909)
  line L2406 (42.6037, 182.909) -> (46.9339, 180.409)
  line L2407 (46.9339, 180.409) -> (51.264, 182.909)
  line L2408 (51.264, 182.909) -> (51.264, 187.909)
  line L2409 (51.264, 187.909) -> (46.9339, 190.409)
  line L2410 (57.5941, 190.409) -> (53.264, 187.909)
  line L2411 (53.264, 187.909) -> (53.264, 182.909)
  line L2412 (53.264, 182.909) -> (57.5941, 180.409)
  line L2413 (57.5941, 180.409) -> (61.9242, 182.909)
  line L2414 (61.9242, 182.909) -> (61.9242, 187.909)
  line L2415 (61.9242, 187.909) -> (57.5941, 190.409)
  line L2416 (68.2544, 190.409) -> (63.9242, 187.909)
  line L2417 (63.9242, 187.909) -> (63.9242, 182.909)
  line L2418 (63.9242, 182.909) -> (68.2544, 180.409)
  line L2419 (68.2544, 180.409) -> (72.5845, 182.909)
  line L2420 (72.5845, 182.909) -> (72.5845, 187.909)
  line L2421 (72.5845, 187.909) -> (68.2544, 190.409)
  line L2422 (78.9146, 190.409) -> (74.5845, 187.909)
  line L2423 (74.5845, 187.909) -> (74.5845, 182.909)
  line L2424 (74.5845, 182.909) -> (78.9146, 180.409)
  line L2425 (78.9146, 180.409) -> (83.2448, 182.909)
  line L2426 (83.2448, 182.909) -> (83.2448, 187.909)
  line L2427 (83.2448, 187.909) -> (78.9146, 190.409)
  line L2428 (89.5749, 190.409) -> (85.2448, 187.909)
  line L2429 (85.2448, 187.909) -> (85.2448, 182.909)
  line L2430 (85.2448, 182.909) -> (89.5749, 180.409)
  line L2431 (89.5749, 180.409) -> (93.905, 182.909)
  line L2432 (93.905, 182.909) -> (93.905, 187.909)
  line L2433 (93.905, 187.909) -> (89.5749, 190.409)
  line L2434 (100.2351, 190.409) -> (95.905, 187.909)
  line L2435 (95.905, 187.909) -> (95.905, 182.909)
  line L2436 (95.905, 182.909) -> (100.2351, 180.409)
  line L2437 (100.2351, 180.409) -> (104.5653, 182.909)
  line L2438 (104.5653, 182.909) -> (104.5653, 187.909)
  line L2439 (104.5653, 187.909) -> (100.2351, 190.409)
  line L2440 (110.8954, 190.409) -> (106.5653, 187.909)
  line L2441 (106.5653, 187.909) -> (106.5653, 182.909)
  line L2442 (106.5653, 182.909) -> (110.8954, 180.409)
  line L2443 (110.8954, 180.409) -> (115.2255, 182.909)
  line L2444 (115.2255, 182.909) -> (115.2255, 187.909)
  line L2445 (115.2255, 187.909) -> (110.8954, 190.409)
  line L2446 (121.5556, 190.409) -> (117.2255, 187.909)
  line L2447 (117.2255, 187.909) -> (117.2255, 182.909)
  line L2448 (117.2255, 182.909) -> (121.5556, 180.409)
  line L2449 (121.5556, 180.409) -> (125.8858, 182.909)
  line L2450 (125.8858, 182.909) -> (125.8858, 187.909)
  line L2451 (125.8858, 187.909) -> (121.5556, 190.409)
  line L2452 (132.2159, 190.409) -> (127.8858, 187.909)
  line L2453 (127.8858, 187.909) -> (127.8858, 182.909)
  line L2454 (127.8858, 182.909) -> (132.2159, 180.409)
  line L2455 (132.2159, 180.409) -> (136.546, 182.909)
  line L2456 (136.546, 182.909) -> (136.546, 187.909)
  line L2457 (136.546, 187.909) -> (132.2159, 190.409)
  line L2458 (142.8762, 190.409) -> (138.546, 187.909)
  line L2459 (138.546, 187.909) -> (138.546, 182.909)
  line L2460 (138.546, 182.909) -> (142.8762, 180.409)
  line L2461 (142.8762, 180.409) -> (147.2063, 182.909)
  line L2462 (147.2063, 182.909) -> (147.2063, 187.909)
  line L2463 (147.2063, 187.909) -> (142.8762, 190.409)
  line L2464 (-64.9988, 199.641) -> (-69.3289, 197.141)
  line L2465 (-69.3289, 197.141) -> (-69.3289, 192.141)
  line L2466 (-69.3289, 192.141) -> (-64.9988, 189.641)
  line L2467 (-64.9988, 189.641) -> (-60.6687, 192.141)
  line L2468 (-60.6687, 192.141) -> (-60.6687, 197.141)
  line L2469 (-60.6687, 197.141) -> (-64.9988, 199.641)
  line L2470 (-54.3385, 199.641) -> (-58.6687, 197.141)
  line L2471 (-58.6687, 197.141) -> (-58.6687, 192.141)
  line L2472 (-58.6687, 192.141) -> (-54.3385, 189.641)
  line L2473 (-54.3385, 189.641) -> (-50.0084, 192.141)
  line L2474 (-50.0084, 192.141) -> (-50.0084, 197.141)
  line L2475 (-50.0084, 197.141) -> (-54.3385, 199.641)
  line L2476 (-43.6783, 199.641) -> (-48.0084, 197.141)
  line L2477 (-48.0084, 197.141) -> (-48.0084, 192.141)
  line L2478 (-48.0084, 192.141) -> (-43.6783, 189.641)
  line L2479 (-43.6783, 189.641) -> (-39.3482, 192.141)
  line L2480 (-39.3482, 192.141) -> (-39.3482, 197.141)
  line L2481 (-39.3482, 197.141) -> (-43.6783, 199.641)
  line L2482 (-33.018, 199.641) -> (-37.3482, 197.141)
  line L2483 (-37.3482, 197.141) -> (-37.3482, 192.141)
  line L2484 (-37.3482, 192.141) -> (-33.018, 189.641)
  line L2485 (-33.018, 189.641) -> (-28.6879, 192.141)
  line L2486 (-28.6879, 192.141) -> (-28.6879, 197.141)
  line L2487 (-28.6879, 197.141) -> (-33.018, 199.641)
  line L2488 (-22.3578, 199.641) -> (-26.6879, 197.141)
  line L2489 (-26.6879, 197.141) -> (-26.6879, 192.141)
  line L2490 (-26.6879, 192.141) -> (-22.3578, 189.641)
  line L2491 (-22.3578, 189.641) -> (-18.0277, 192.141)
  line L2492 (-18.0277, 192.141) -> (-18.0277, 197.141)
  line L2493 (-18.0277, 197.141) -> (-22.3578, 199.641)
  line L2494 (-11.6975, 199.641) -> (-16.0277, 197.141)
  line L2495 (-16.0277, 197.141) -> (-16.0277, 192.141)
  line L2496 (-16.0277, 192.141) -> (-11.6975, 189.641)
  line L2497 (-11.6975, 189.641) -> (-7.3674, 192.141)
  line L2498 (-7.3674, 192.141) -> (-7.3674, 197.141)
  line L2499 (-7.3674, 197.141) -> (-11.6975, 199.641)
  line L2500 (-1.0373, 199.641) -> (-5.3674, 197.141)
  line L2501 (-5.3674, 197.141) -> (-5.3674, 192.141)
  line L2502 (-5.3674, 192.141) -> (-1.0373, 189.641)
  line L2503 (-1.0373, 189.641) -> (3.2929, 192.141)
  line L2504 (3.2929, 192.141) -> (3.2929, 197.141)
  line L2505 (3.2929, 197.141) -> (-1.0373, 199.641)
  line L2506 (9.623, 199.641) -> (5.2929, 197.141)
  line L2507 (5.2929, 197.141) -> (5.2929, 192.141)
  line L2508 (5.2929, 192.141) -> (9.623, 189.641)
  line L2509 (9.623, 189.641) -> (13.9531, 192.141)
  line L2510 (13.9531, 192.141) -> (13.9531, 197.141)
  line L2511 (13.9531, 197.141) -> (9.623, 199.641)
  line L2512 (20.2832, 199.641) -> (15.9531, 197.141)
  line L2513 (15.9531, 197.141) -> (15.9531, 192.141)
  line L2514 (15.9531, 192.141) -> (20.2832, 189.641)
  line L2515 (20.2832, 189.641) -> (24.6134, 192.141)
  line L2516 (24.6134, 192.141) -> (24.6134, 197.141)
  line L2517 (24.6134, 197.141) -> (20.2832, 199.641)
  line L2518 (30.9435, 199.641) -> (26.6134, 197.141)
  line L2519 (26.6134, 197.141) -> (26.6134, 192.141)
  line L2520 (26.6134, 192.141) -> (30.9435, 189.641)
  line L2521 (30.9435, 189.641) -> (35.2736, 192.141)
  line L2522 (35.2736, 192.141) -> (35.2736, 197.141)
  line L2523 (35.2736, 197.141) -> (30.9435, 199.641)
  line L2524 (41.6037, 199.641) -> (37.2736, 197.141)
  line L2525 (37.2736, 197.141) -> (37.2736, 192.141)
  line L2526 (37.2736, 192.141) -> (41.6037, 189.641)
  line L2527 (41.6037, 189.641) -> (45.9339, 192.141)
  line L2528 (45.9339, 192.141) -> (45.9339, 197.141)
  line L2529 (45.9339, 197.141) -> (41.6037, 199.641)
  line L2530 (52.264, 199.641) -> (47.9339, 197.141)
  line L2531 (47.9339, 197.141) -> (47.9339, 192.141)
  line L2532 (47.9339, 192.141) -> (52.264, 189.641)
  line L2533 (52.264, 189.641) -> (56.5941, 192.141)
  line L2534 (56.5941, 192.141) -> (56.5941, 197.141)
  line L2535 (56.5941, 197.141) -> (52.264, 199.641)
  line L2536 (62.9242, 199.641) -> (58.5941, 197.141)
  line L2537 (58.5941, 197.141) -> (58.5941, 192.141)
  line L2538 (58.5941, 192.141) -> (62.9242, 189.641)
  line L2539 (62.9242, 189.641) -> (67.2544, 192.141)
  line L2540 (67.2544, 192.141) -> (67.2544, 197.141)
  line L2541 (67.2544, 197.141) -> (62.9242, 199.641)
  line L2542 (73.5845, 199.641) -> (69.2544, 197.141)
  line L2543 (69.2544, 197.141) -> (69.2544, 192.141)
  line L2544 (69.2544, 192.141) -> (73.5845, 189.641)
  line L2545 (73.5845, 189.641) -> (77.9146, 192.141)
  line L2546 (77.9146, 192.141) -> (77.9146, 197.141)
  line L2547 (77.9146, 197.141) -> (73.5845, 199.641)
  line L2548 (84.2448, 199.641) -> (79.9146, 197.141)
  line L2549 (79.9146, 197.141) -> (79.9146, 192.141)
  line L2550 (79.9146, 192.141) -> (84.2448, 189.641)
  line L2551 (84.2448, 189.641) -> (88.5749, 192.141)
  line L2552 (88.5749, 192.141) -> (88.5749, 197.141)
  line L2553 (88.5749, 197.141) -> (84.2448, 199.641)
  line L2554 (94.905, 199.641) -> (90.5749, 197.141)
  line L2555 (90.5749, 197.141) -> (90.5749, 192.141)
  line L2556 (90.5749, 192.141) -> (94.905, 189.641)
  line L2557 (94.905, 189.641) -> (99.2351, 192.141)
  line L2558 (99.2351, 192.141) -> (99.2351, 197.141)
  line L2559 (99.2351, 197.141) -> (94.905, 199.641)
  line L2560 (105.5653, 199.641) -> (101.2351, 197.141)
  line L2561 (101.2351, 197.141) -> (101.2351, 192.141)
  line L2562 (101.2351, 192.141) -> (105.5653, 189.641)
  line L2563 (105.5653, 189.641) -> (109.8954, 192.141)
  line L2564 (109.8954, 192.141) -> (109.8954, 197.141)
  line L2565 (109.8954, 197.141) -> (105.5653, 199.641)
  line L2566 (116.2255, 199.641) -> (111.8954, 197.141)
  line L2567 (111.8954, 197.141) -> (111.8954, 192.141)
  line L2568 (111.8954, 192.141) -> (116.2255, 189.641)
  line L2569 (116.2255, 189.641) -> (120.5556, 192.141)
  line L2570 (120.5556, 192.141) -> (120.5556, 197.141)
  line L2571 (120.5556, 197.141) -> (116.2255, 199.641)
  line L2572 (126.8858, 199.641) -> (122.5556, 197.141)
  line L2573 (122.5556, 197.141) -> (122.5556, 192.141)
  line L2574 (122.5556, 192.141) -> (126.8858, 189.641)
  line L2575 (126.8858, 189.641) -> (131.2159, 192.141)
  line L2576 (131.2159, 192.141) -> (131.2159, 197.141)
  line L2577 (131.2159, 197.141) -> (126.8858, 199.641)
  line L2578 (137.546, 199.641) -> (133.2159, 197.141)
  line L2579 (133.2159, 197.141) -> (133.2159, 192.141)
  line L2580 (133.2159, 192.141) -> (137.546, 189.641)
  line L2581 (137.546, 189.641) -> (141.8762, 192.141)
  line L2582 (141.8762, 192.141) -> (141.8762, 197.141)
  line L2583 (141.8762, 197.141) -> (137.546, 199.641)
  line L2584 (148.2063, 199.641) -> (143.8762, 197.141)
  line L2585 (143.8762, 197.141) -> (143.8762, 192.141)
  line L2586 (143.8762, 192.141) -> (148.2063, 189.641)
  line L2587 (148.2063, 189.641) -> (152.5364, 192.141)
  line L2588 (152.5364, 192.141) -> (152.5364, 197.141)
  line L2589 (152.5364, 197.141) -> (148.2063, 199.641)
  line L2590 (-59.6687, 208.8731) -> (-63.9988, 206.3731)
  line L2591 (-63.9988, 206.3731) -> (-63.9988, 201.3731)
  line L2592 (-63.9988, 201.3731) -> (-59.6687, 198.8731)
  line L2593 (-59.6687, 198.8731) -> (-55.3385, 201.3731)
  line L2594 (-55.3385, 201.3731) -> (-55.3385, 206.3731)
  line L2595 (-55.3385, 206.3731) -> (-59.6687, 208.8731)
  line L2596 (-49.0084, 208.8731) -> (-53.3385, 206.3731)
  line L2597 (-53.3385, 206.3731) -> (-53.3385, 201.3731)
  line L2598 (-53.3385, 201.3731) -> (-49.0084, 198.8731)
  line L2599 (-49.0084, 198.8731) -> (-44.6783, 201.3731)
  line L2600 (-44.6783, 201.3731) -> (-44.6783, 206.3731)
  line L2601 (-44.6783, 206.3731) -> (-49.0084, 208.8731)
  line L2602 (-38.3482, 208.8731) -> (-42.6783, 206.3731)
  line L2603 (-42.6783, 206.3731) -> (-42.6783, 201.3731)
  line L2604 (-42.6783, 201.3731) -> (-38.3482, 198.8731)
  line L2605 (-38.3482, 198.8731) -> (-34.018, 201.3731)
  line L2606 (-34.018, 201.3731) -> (-34.018, 206.3731)
  line L2607 (-34.018, 206.3731) -> (-38.3482, 208.8731)
  line L2608 (-27.6879, 208.8731) -> (-32.018, 206.3731)
  line L2609 (-32.018, 206.3731) -> (-32.018, 201.3731)
  line L2610 (-32.018, 201.3731) -> (-27.6879, 198.8731)
  line L2611 (-27.6879, 198.8731) -> (-23.3578, 201.3731)
  line L2612 (-23.3578, 201.3731) -> (-23.3578, 206.3731)
  line L2613 (-23.3578, 206.3731) -> (-27.6879, 208.8731)
  line L2614 (-17.0277, 208.8731) -> (-21.3578, 206.3731)
  line L2615 (-21.3578, 206.3731) -> (-21.3578, 201.3731)
  line L2616 (-21.3578, 201.3731) -> (-17.0277, 198.8731)
  line L2617 (-17.0277, 198.8731) -> (-12.6975, 201.3731)
  line L2618 (-12.6975, 201.3731) -> (-12.6975, 206.3731)
  line L2619 (-12.6975, 206.3731) -> (-17.0277, 208.8731)
  line L2620 (-6.3674, 208.8731) -> (-10.6975, 206.3731)
  line L2621 (-10.6975, 206.3731) -> (-10.6975, 201.3731)
  line L2622 (-10.6975, 201.3731) -> (-6.3674, 198.8731)
  line L2623 (-6.3674, 198.8731) -> (-2.0373, 201.3731)
  line L2624 (-2.0373, 201.3731) -> (-2.0373, 206.3731)
  line L2625 (-2.0373, 206.3731) -> (-6.3674, 208.8731)
  line L2626 (4.2929, 208.8731) -> (-0.0373, 206.3731)
  line L2627 (-0.0373, 206.3731) -> (-0.0373, 201.3731)
  line L2628 (-0.0373, 201.3731) -> (4.2929, 198.8731)
  line L2629 (4.2929, 198.8731) -> (8.623, 201.3731)
  line L2630 (8.623, 201.3731) -> (8.623, 206.3731)
  line L2631 (8.623, 206.3731) -> (4.2929, 208.8731)
  line L2632 (14.9531, 208.8731) -> (10.623, 206.3731)
  line L2633 (10.623, 206.3731) -> (10.623, 201.3731)
  line L2634 (10.623, 201.3731) -> (14.9531, 198.8731)
  line L2635 (14.9531, 198.8731) -> (19.2832, 201.3731)
  line L2636 (19.2832, 201.3731) -> (19.2832, 206.3731)
  line L2637 (19.2832, 206.3731) -> (14.9531, 208.8731)
  line L2638 (25.6134, 208.8731) -> (21.2832, 206.3731)
  line L2639 (21.2832, 206.3731) -> (21.2832, 201.3731)
  line L2640 (21.2832, 201.3731) -> (25.6134, 198.8731)
  line L2641 (25.6134, 198.8731) -> (29.9435, 201.3731)
  line L2642 (29.9435, 201.3731) -> (29.9435, 206.3731)
  line L2643 (29.9435, 206.3731) -> (25.6134, 208.8731)
  line L2644 (36.2736, 208.8731) -> (31.9435, 206.3731)
  line L2645 (31.9435, 206.3731) -> (31.9435, 201.3731)
  line L2646 (31.9435, 201.3731) -> (36.2736, 198.8731)
  line L2647 (36.2736, 198.8731) -> (40.6037, 201.3731)
  line L2648 (40.6037, 201.3731) -> (40.6037, 206.3731)
  line L2649 (40.6037, 206.3731) -> (36.2736, 208.8731)
  line L2650 (46.9339, 208.8731) -> (42.6037, 206.3731)
  line L2651 (42.6037, 206.3731) -> (42.6037, 201.3731)
  line L2652 (42.6037, 201.3731) -> (46.9339, 198.8731)
  line L2653 (46.9339, 198.8731) -> (51.264, 201.3731)
  line L2654 (51.264, 201.3731) -> (51.264, 206.3731)
  line L2655 (51.264, 206.3731) -> (46.9339, 208.8731)
  line L2656 (57.5941, 208.8731) -> (53.264, 206.3731)
  line L2657 (53.264, 206.3731) -> (53.264, 201.3731)
  line L2658 (53.264, 201.3731) -> (57.5941, 198.8731)
  line L2659 (57.5941, 198.8731) -> (61.9242, 201.3731)
  line L2660 (61.9242, 201.3731) -> (61.9242, 206.3731)
  line L2661 (61.9242, 206.3731) -> (57.5941, 208.8731)
  line L2662 (68.2544, 208.8731) -> (63.9242, 206.3731)
  line L2663 (63.9242, 206.3731) -> (63.9242, 201.3731)
  line L2664 (63.9242, 201.3731) -> (68.2544, 198.8731)
  line L2665 (68.2544, 198.8731) -> (72.5845, 201.3731)
  line L2666 (72.5845, 201.3731) -> (72.5845, 206.3731)
  line L2667 (72.5845, 206.3731) -> (68.2544, 208.8731)
  line L2668 (78.9146, 208.8731) -> (74.5845, 206.3731)
  line L2669 (74.5845, 206.3731) -> (74.5845, 201.3731)
  line L2670 (74.5845, 201.3731) -> (78.9146, 198.8731)
  line L2671 (78.9146, 198.8731) -> (83.2448, 201.3731)
  line L2672 (83.2448, 201.3731) -> (83.2448, 206.3731)
  line L2673 (83.2448, 206.3731) -> (78.9146, 208.8731)
  line L2674 (89.5749, 208.8731) -> (85.2448, 206.3731)
  line L2675 (85.2448, 206.3731) -> (85.2448, 201.3731)
  line L2676 (85.2448, 201.3731) -> (89.5749, 198.8731)
  line L2677 (89.5749, 198.8731) -> (93.905, 201.3731)
  line L2678 (93.905, 201.3731) -> (93.905, 206.3731)
  line L2679 (93.905, 206.3731) -> (89.5749, 208.8731)
  line L2680 (100.2351, 208.8731) -> (95.905, 206.3731)
  line L2681 (95.905, 206.3731) -> (95.905, 201.3731)
  line L2682 (95.905, 201.3731) -> (100.2351, 198.8731)
  line L2683 (100.2351, 198.8731) -> (104.5653, 201.3731)
  line L2684 (104.5653, 201.3731) -> (104.5653, 206.3731)
  line L2685 (104.5653, 206.3731) -> (100.2351, 208.8731)
  line L2686 (110.8954, 208.8731) -> (106.5653, 206.3731)
  line L2687 (106.5653, 206.3731) -> (106.5653, 201.3731)
  line L2688 (106.5653, 201.3731) -> (110.8954, 198.8731)
  line L2689 (110.8954, 198.8731) -> (115.2255, 201.3731)
  line L2690 (115.2255, 201.3731) -> (115.2255, 206.3731)
  line L2691 (115.2255, 206.3731) -> (110.8954, 208.8731)
  line L2692 (121.5556, 208.8731) -> (117.2255, 206.3731)
  line L2693 (117.2255, 206.3731) -> (117.2255, 201.3731)
  line L2694 (117.2255, 201.3731) -> (121.5556, 198.8731)
  line L2695 (121.5556, 198.8731) -> (125.8858, 201.3731)
  line L2696 (125.8858, 201.3731) -> (125.8858, 206.3731)
  line L2697 (125.8858, 206.3731) -> (121.5556, 208.8731)
  line L2698 (132.2159, 208.8731) -> (127.8858, 206.3731)
  line L2699 (127.8858, 206.3731) -> (127.8858, 201.3731)
  line L2700 (127.8858, 201.3731) -> (132.2159, 198.8731)
  line L2701 (132.2159, 198.8731) -> (136.546, 201.3731)
  line L2702 (136.546, 201.3731) -> (136.546, 206.3731)
  line L2703 (136.546, 206.3731) -> (132.2159, 208.8731)
  line L2704 (142.8762, 208.8731) -> (138.546, 206.3731)
  line L2705 (138.546, 206.3731) -> (138.546, 201.3731)
  line L2706 (138.546, 201.3731) -> (142.8762, 198.8731)
  line L2707 (142.8762, 198.8731) -> (147.2063, 201.3731)
  line L2708 (147.2063, 201.3731) -> (147.2063, 206.3731)
  line L2709 (147.2063, 206.3731) -> (142.8762, 208.8731)
  line L2710 (-64.9988, 218.1051) -> (-69.3289, 215.6051)
  line L2711 (-69.3289, 215.6051) -> (-69.3289, 210.6051)
  line L2712 (-69.3289, 210.6051) -> (-64.9988, 208.1051)
  line L2713 (-64.9988, 208.1051) -> (-60.6687, 210.6051)
  line L2714 (-60.6687, 210.6051) -> (-60.6687, 215.6051)
  line L2715 (-60.6687, 215.6051) -> (-64.9988, 218.1051)
  line L2716 (-54.3385, 218.1051) -> (-58.6687, 215.6051)
  line L2717 (-58.6687, 215.6051) -> (-58.6687, 210.6051)
  line L2718 (-58.6687, 210.6051) -> (-54.3385, 208.1051)
  line L2719 (-54.3385, 208.1051) -> (-50.0084, 210.6051)
  line L2720 (-50.0084, 210.6051) -> (-50.0084, 215.6051)
  line L2721 (-50.0084, 215.6051) -> (-54.3385, 218.1051)
  line L2722 (-43.6783, 218.1051) -> (-48.0084, 215.6051)
  line L2723 (-48.0084, 215.6051) -> (-48.0084, 210.6051)
  line L2724 (-48.0084, 210.6051) -> (-43.6783, 208.1051)
  line L2725 (-43.6783, 208.1051) -> (-39.3482, 210.6051)
  line L2726 (-39.3482, 210.6051) -> (-39.3482, 215.6051)
  line L2727 (-39.3482, 215.6051) -> (-43.6783, 218.1051)
  line L2728 (-33.018, 218.1051) -> (-37.3482, 215.6051)
  line L2729 (-37.3482, 215.6051) -> (-37.3482, 210.6051)
  line L2730 (-37.3482, 210.6051) -> (-33.018, 208.1051)